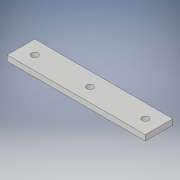
# Autodesk Inventor part: 1
Saved by Autodesk Inventor 2019 (Build 230136000, 136)
## iProperties
Created: 2021-01-29
Part Number: 1
Material: 一般
Document SubType Name: Modeling
Designer: X1 Carbon
Density: 1 g/cm^3
Appearance: 既定
Author: X1 Carbon
Autodesk Inventor part; units mm, degrees
ref_plane "YZ Plane" through (0, 0, 0) normal (1, 0, 0) x (0, 1, 0)
ref_plane "XZ Plane" through (0, 0, 0) normal (0, 1, 0) x (-1, 0, 0)
ref_plane "XY Plane" through (0, 0, 0) normal (0, 0, 1) x (1, 0, 0)
sketch "スケッチ1" plane through (0, 0, 0) normal (0, 1, 0) x (-1, 0, 0)
  circle A0 centre (0, 0) radius 1.75
  circle A1 centre (30, 0) radius 1.75
  circle A2 centre (-30, 0) radius 1.75
  line L0 (-37.5, 7.5) -> (37.5, 7.5)
  line L1 (37.5, 7.5) -> (37.5, -7.5)
  line L2 (37.5, -7.5) -> (-37.5, -7.5)
  line L3 (-37.5, -7.5) -> (-37.5, 7.5)
  line L4 (-37.5, 7.5) -> (37.5, -7.5) construction
  line L5 (37.5, 7.5) -> (-37.5, -7.5) construction
  line L6 (-37.5, 7.5) -> (37.5, 7.5) construction
  dimension "d0" = 3.5
  dimension "d1" = 3.5
  dimension "d2" = 3.5
  dimension "d3" = 75
  dimension "d4" = 0
  dimension "d5" = 15
  constraints: 14 end point, 3 centre point, 2 horizontal, 2 midpoint, 2 parallel, 1 coincident, 1 collinear, 1 perpendicular
  measures "d0" diameter of A0
  measures "d1" diameter of A1
  measures "d2" diameter of A2
  measures "d3" distance of L0.start L0.end
  measures "d4" distance between parallel lines of L0 L6
  measures "d5" distance of L0.end L1.end
extrude "押し出し1" add sketch "スケッチ1" along normal blind 3
